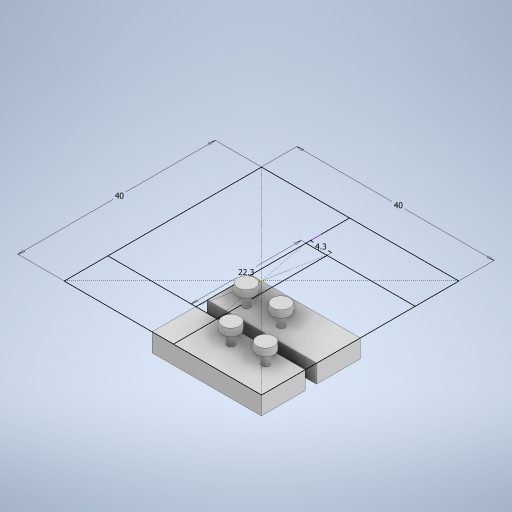
# Autodesk Inventor part: top-small
Saved by Autodesk Inventor 2023 (Build 270158000, 158)
## iProperties
Created: 2023-08-09
Part Number: top-small
Material: Generic
Document SubType Name: Modeling
Designer: AxLab
Density: 1 g/cm^3
Appearance: Default
Author: AxLab
Autodesk Inventor part; units mm, degrees
ref_plane "YZ Plane" through (0, 0, 0) normal (1, 0, 0) x (0, 1, 0)
ref_plane "XZ Plane" through (0, 0, 0) normal (0, 1, 0) x (-1, 0, 0)
ref_plane "XY Plane" through (0, 0, 0) normal (0, 0, 1) x (1, 0, 0)
sketch "Sketch1" plane through (0, 0, 0) normal (0, 1, 0) x (-1, 0, 0)
  line L0 (-2.15, 11.15) -> (2.15, 11.15)
  line L1 (2.15, 11.15) -> (2.15, -11.15)
  line L2 (2.15, -11.15) -> (-2.15, -11.15)
  line L3 (-2.15, -11.15) -> (-2.15, 11.15)
  line L4 (-2.15, 11.15) -> (2.15, -11.15) construction
  line L5 (2.15, 11.15) -> (-2.15, -11.15) construction
  line L6 (-20, 20) -> (20, 20)
  line L7 (20, 20) -> (20, -20)
  line L8 (20, -20) -> (-20, -20)
  line L9 (-20, -20) -> (-20, 20)
  line L10 (-20, 20) -> (20, -20) construction
  line L11 (20, 20) -> (-20, -20) construction
  line L12 (2.15, -11.15) -> (-20, -11.15)
  line L13 (2.15, 11.15) -> (2.15, -20)
  line L14 (-2.15, 11.15) -> (20, 11.15)
  line L15 (-2.15, -11.15) -> (-2.15, 20)
  line L16 (2.15, -11.15) -> (-0.85, -11.15)
  line L17 (2.15, -14.15) -> (2.15, -11.15)
  point P0 (0, 0)
  dimension "d0" = 4.3
  dimension "d1" = 22.3
  dimension "d2" = 40
  dimension "d3" = 40
  constraints: 36 end point, 5 point on line, 4 midpoint, 4 parallel, 4 perpendicular, 3 horizontal, 1 vertical
  measures "d0" distance of L1.end L2.end
  measures "d1" distance of L0.end L1.end
  measures "d2" distance of L7.end L8.end
  measures "d3" distance of L6.end L7.end
extrude "Extrusion1" add sketch "Sketch1" along normal blind 3.7 contours L15 L6 L7 L14 L0 | L2 L13 L8 L9 L12
sketch "Sketch6" plane through (0, 0, 0) normal (0, 1, 0) x (-1, 0, 0)
  line L0 (-20, -16.15) -> (-20, -11.15)
  circle A0 centre (-15, -14.15) radius 0.75
  circle A1 centre (-8, -14.15) radius 0.75
  line L1 (-2.15, 11.15) -> (20, 11.15) projected
  circle A2 centre (15, 14.15) radius 0.75
  circle A3 centre (8, 14.15) radius 0.75
  point P0 (0, 0)
  dimension "d58" = 1.5
  dimension "d59" = 1.5
  dimension "d64" = 1.5
  dimension "d76" = 1.5
  constraints: 4 centre point, 2 end point
  measures "d58" diameter of A0
  measures "d59" diameter of A1
  measures "d64" diameter of A2
  measures "d76" diameter of A3
extrude "Extrusion5" add sketch "Sketch6" against normal blind 2.5
sketch "Sketch9" plane through (15, -2.5, -14.15) normal (0, -1, 0) x (1, 0, 0)
  circle A0 centre (0, 0) radius 0.75 projected
  circle A1 centre (0, 0) radius 1.75
  circle A2 centre (-7, 0) radius 0.75 projected
  circle A3 centre (-7, 0) radius 1.75
  circle A4 centre (-23, 28.3) radius 0.75 projected
  circle A5 centre (-23, 28.3) radius 1.75
  circle A6 centre (-30, 28.3) radius 0.75 projected
  circle A7 centre (-30, 28.3) radius 1.75
  point P0 (-15, 14.15)
  dimension "d77" = 3.5
  dimension "d78" = 3.5
  dimension "d79" = 3.5
  dimension "d80" = 3.5
  constraints: 4 centre point, 4 coincident
  measures "d77" diameter of A1
  measures "d78" diameter of A3
  measures "d79" diameter of A5
  measures "d80" diameter of A7
extrude "Extrusion8" add sketch "Sketch9" along normal blind 1.5 contours A0 | A1 | A2 | A3 | A4 | A5 | A6 | A7
move or copy body "Move Body1" bodies to move or copy 1 copy no rotation origin (0, 0, 0) rotation axis (0, 0, 1) rotation angle 180
split body "Split1" sketch "Sketch1" result two bodies curves L14 first body at (6.6667, -3.2, 17.05)
move or copy body "Move Body2" bodies to move or copy 3 copy no translate (17.85, 0, 20)
body "Solid4"
body "Solid5"
